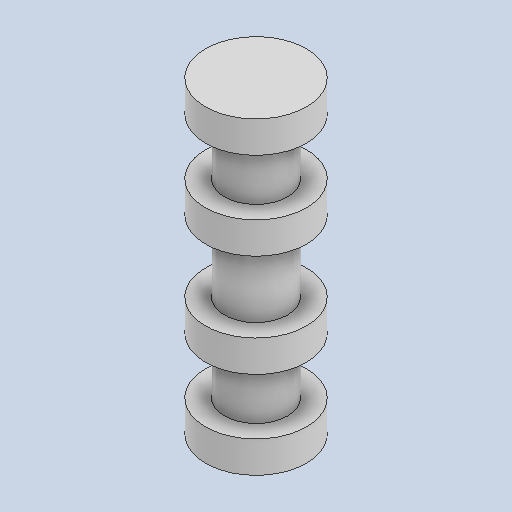
# Autodesk Inventor part: Wrist Pin
Saved by Autodesk Inventor 2023 (Build 270158000, 158)
## iProperties
Created: 2022-10-29
Part Number: Wrist Pin
Material: Generic
Document SubType Name: Modeling
Designer: tommy
Density: 1 g/cm^3
Appearance: Default
Mass: 1.61282 g
Surface Area: 12.313 cm^2
Volume: 1.61282 cm^3
Author: tommy
Autodesk Inventor part; units mm, degrees
ref_plane "YZ Plane" through (0, 0, 0) normal (1, 0, 0) x (0, 1, 0)
ref_plane "XZ Plane" through (0, 0, 0) normal (0, 1, 0) x (-1, 0, 0)
ref_plane "XY Plane" through (0, 0, 0) normal (0, 0, 1) x (1, 0, 0)
sketch "Sketch1" plane through (0, 0, 0) normal (0, 0, 1) x (1, 0, 0)
  line L0 (0, 0) -> (0, 31.115)
  line L1 (0, 31.115) -> (5.08, 31.115)
  line L2 (5.08, 31.115) -> (5.08, 27.94)
  line L3 (5.08, 27.94) -> (3.175, 27.94)
  line L4 (3.175, 15.5575) -> (3.175, 19.1294)
  line L5 (3.175, 19.1294) -> (5.08, 19.1294)
  line L6 (5.08, 19.1294) -> (5.08, 22.3044)
  line L7 (5.08, 22.3044) -> (3.175, 22.3044)
  line L8 (3.175, 15.5575) -> (3.175, 19.1294)
  line L9 (3.175, 22.3044) -> (3.175, 27.94)
  line L10 (0, 0) -> (5.08, 0)
  line L11 (5.08, 0) -> (5.08, 3.175)
  line L12 (5.08, 3.175) -> (3.175, 3.175)
  line L13 (3.175, 15.5575) -> (3.175, 11.9856)
  line L14 (3.175, 11.9856) -> (5.08, 11.9856)
  line L15 (5.08, 11.9856) -> (5.08, 8.8106)
  line L16 (5.08, 8.8106) -> (3.175, 8.8106)
  line L17 (3.175, 15.5575) -> (3.175, 11.9856)
  line L18 (3.175, 8.8106) -> (3.175, 3.175)
  dimension "d0" = 31.115
  dimension "d1" = 5.08
  dimension "d2" = 3.175
  dimension "d5" = 3.175
  constraints: 38 end point, 4 perpendicular, 2 horizontal, 1 vertical
  measures "d0" distance of L0.start L0.end
  measures "d1" distance of L0.end L1.end
  measures "d2" distance of L1.end L2.end
  measures "d5" distance of L5.end L6.end
revolve "Revolution1" add sketch "Sketch1" angle 360 about axis through (0, 0, 0) along (0, 1, 0)
body "Solid1"
